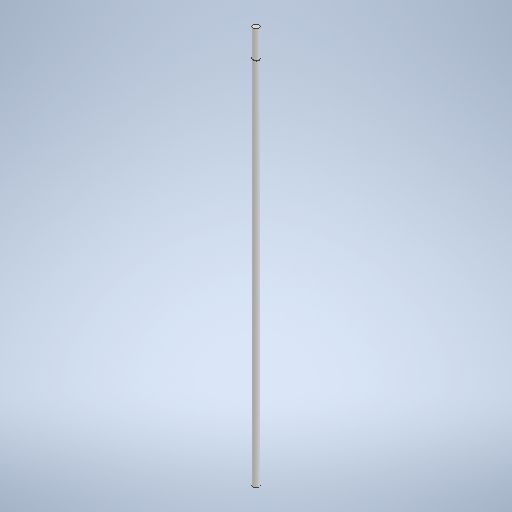
# Autodesk Inventor part: Вал
Saved by Autodesk Inventor 2025 (Build 290162010, 162A)
## iProperties
Created: 2024-04-09
Part Number: Вал
Material: Generic
Document SubType Name: Modeling
Designer: pokla
Density: 1 g/cm^3
Appearance: Default
Author: pokla
Autodesk Inventor part; units mm, degrees
ref_plane "YZ Plane" through (0, 0, 0) normal (1, 0, 0) x (0, 1, 0)
ref_plane "XZ Plane" through (0, 0, 0) normal (0, 1, 0) x (-1, 0, 0)
ref_plane "XY Plane" through (0, 0, 0) normal (0, 0, 1) x (1, 0, 0)
sketch "Sketch1" plane through (0, 0, 0) normal (1, 0, 0) x (0, 1, 0)
  line L0 (550, 0) -> (-550, 0)
  line L1 (-550, 0) -> (-550, -8.5)
  line L2 (-550, -8.5) -> (550, -8.5)
  line L3 (550, -8.5) -> (550, 0)
  line L4 (474, -8.5) -> (474, -7.5)
  line L5 (474, -7.5) -> (473, -7.5)
  line L6 (473, -7.5) -> (473, -8.5)
  point P0 (0, 0)
  point P1 (0, 0)
  dimension "d0" = 1100
  dimension "d1" = 8.5
  dimension "d2" = 1
  dimension "d3" = 1
  dimension "d4" = 76
  constraints: 14 end point, 3 perpendicular, 2 parallel, 2 point on line, 1 coincident, 1 horizontal, 1 midpoint, 1 vertical
  measures "d0" distance of L2.end L1.end
  measures "d1" distance of L1.end L0.end
  measures "d2" distance of L4.start L4.end
  measures "d3" distance of L4.end L5.end
  measures "d4" distance between parallel lines of L3 L4
revolve "Revolution1" add sketch "Sketch1" angle 360 about axis through (0, 550, 0) along (0, -1, 0) contours L3 L2 L4 L5 L6 L1 L0
body "Solid1"
